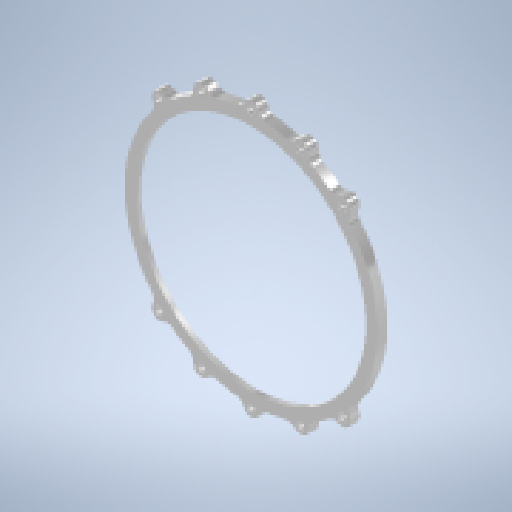
# Autodesk Inventor part: 出力ベアリング抑え
Saved by Autodesk Inventor 2024 (Build 280153000, 153)
## iProperties
Created: 2023-05-29
Part Number: 出力ベアリング抑え
Material: アルミニウム 6061
Document SubType Name: Modeling
Designer: yuta2
Density: 2.7 g/cm^3
Appearance: アルミニウム - フラット
Author: yuta2
Autodesk Inventor part; units mm, degrees
ref_plane "YZ Plane" through (0, 0, 0) normal (1, 0, 0) x (0, 1, 0)
ref_plane "XZ Plane" through (0, 0, 0) normal (0, 1, 0) x (-1, 0, 0)
ref_plane "XY Plane" through (0, 0, 0) normal (0, 0, 1) x (1, 0, 0)
sketch "スケッチ1" plane through (0, 0, 0) normal (0, 0, 1) x (1, 0, 0)
  circle A0 centre (0, 0) radius 59
  circle A1 centre (0, 0) radius 65
  dimension "d0" = 118
  dimension "d1" = 130
  constraints: 2 centre point, 2 coincident
  measures "d0" diameter of A0
  measures "d1" diameter of A1
extrude "押し出し1" add sketch "スケッチ1" along normal blind 2.5
sketch "スケッチ2" plane through (0, 0, 0) normal (0, 0, -1) x (-1, 0, 0)
  circle A0 centre (0, 0) radius 65 projected
  circle A1 centre (0, 0) radius 59 projected
  circle A2 centre (0, 0) radius 62.5
  dimension "d4" = 125
  constraints: 1 centre point, 1 coincident
  measures "d4" diameter of A2
extrude "押し出し2" add sketch "スケッチ2" along normal blind 2.5 contours A0
sketch "スケッチ3" plane through (0, 0, 2.5) normal (0, 0, 1) x (1, 0, 0)
  circle A0 centre (0, 0) radius 65 projected
  circle A1 centre (0, 0) radius 62.5 projected
  circle A2 centre (0, 66.5) radius 4
  point P0 (3.6646, 64.8966)
  point P1 (-3.6646, 64.8966)
  dimension "d7" = 8
  constraints: 1 centre point, 1 tangent, 1 vertical alignment
  measures "d7" diameter of A2
extrude "押し出し3" add sketch "スケッチ3" against normal blind 5 contours A0 A2 picked at (-0.1169, 66.8205)
fillet "フィレット1" radius 5 4 edges at (3.6646, 64.8966, 1.25) (3.6646, 64.8966, -1.25) (-3.6646, 64.8966, 1.25) (-3.6646, 64.8966, -1.25)
pattern_circular "円形状パターン1" count 16 over 360 about axis through (0, 0, 0) along (0, 0, 1) of "押し出し3", "フィレット1"
sketch "スケッチ4" plane through (0, 0, 2.5) normal (0, 0, 1) x (1, 0, 0)
  arc A0 (-7.8847, 64.52) -> (-17.4062, 62.6261) centre (0, 0) ccw projected
  arc A1 (-22.4692, 64.1071) -> (-17.4062, 62.6261) centre (-18.7451, 67.4435) ccw projected
  arc A2 (-22.4692, 64.1071) -> (-29.4424, 61.2187) centre (-25.4484, 61.438) ccw projected
  arc A3 (-31.9753, 56.5914) -> (-29.4424, 61.2187) centre (-34.4349, 60.9445) ccw projected
  arc A4 (-31.9753, 56.5914) -> (-40.0472, 51.1979) centre (0, 0) ccw projected
  arc A5 (-45.2916, 50.6286) -> (-40.0472, 51.1979) centre (-43.1277, 55.1362) ccw projected
  arc A6 (-45.2916, 50.6286) -> (-50.6286, 45.2916) centre (-47.0226, 47.0226) ccw projected
  arc A7 (-51.1979, 40.0472) -> (-50.6286, 45.2916) centre (-55.1362, 43.1277) ccw projected
  arc A8 (-51.1979, 40.0472) -> (-56.5914, 31.9753) centre (0, 0) ccw projected
  arc A9 (-61.2187, 29.4424) -> (-56.5914, 31.9753) centre (-60.9445, 34.4349) ccw projected
  arc A10 (-61.2187, 29.4424) -> (-64.1071, 22.4692) centre (-61.438, 25.4484) ccw projected
  arc A11 (-62.6261, 17.4062) -> (-64.1071, 22.4692) centre (-67.4435, 18.7451) ccw projected
  arc A12 (-62.6261, 17.4062) -> (-64.52, 7.8847) centre (0, 0) ccw projected
  arc A13 (-67.8258, 3.7739) -> (-64.52, 7.8847) centre (-69.4831, 8.4912) ccw projected
  arc A14 (-67.8258, 3.7739) -> (-67.8258, -3.7739) centre (-66.5, 0) ccw projected
  arc A15 (-64.52, -7.8847) -> (-67.8258, -3.7739) centre (-69.4831, -8.4912) ccw projected
  arc A16 (-64.52, -7.8847) -> (-62.6261, -17.4062) centre (0, 0) ccw projected
  arc A17 (-64.1071, -22.4692) -> (-62.6261, -17.4062) centre (-67.4435, -18.7451) ccw projected
  arc A18 (-64.1071, -22.4692) -> (-61.2187, -29.4424) centre (-61.438, -25.4484) ccw projected
  arc A19 (-56.5914, -31.9753) -> (-61.2187, -29.4424) centre (-60.9445, -34.4349) ccw projected
  arc A20 (-56.5914, -31.9753) -> (-51.1979, -40.0472) centre (0, 0) ccw projected
  arc A21 (-50.6286, -45.2916) -> (-51.1979, -40.0472) centre (-55.1362, -43.1277) ccw projected
  arc A22 (-50.6286, -45.2916) -> (-45.2916, -50.6286) centre (-47.0226, -47.0226) ccw projected
  arc A23 (-40.0472, -51.1979) -> (-45.2916, -50.6286) centre (-43.1277, -55.1362) ccw projected
  arc A24 (-40.0472, -51.1979) -> (-31.9753, -56.5914) centre (0, 0) ccw projected
  arc A25 (-29.4424, -61.2187) -> (-31.9753, -56.5914) centre (-34.4349, -60.9445) ccw projected
  arc A26 (-29.4424, -61.2187) -> (-22.4692, -64.1071) centre (-25.4484, -61.438) ccw projected
  arc A27 (-17.4062, -62.6261) -> (-22.4692, -64.1071) centre (-18.7451, -67.4435) ccw projected
  arc A28 (-17.4062, -62.6261) -> (-7.8847, -64.52) centre (0, 0) ccw projected
  arc A29 (-3.7739, -67.8258) -> (-7.8847, -64.52) centre (-8.4912, -69.4831) ccw projected
  arc A30 (-3.7739, -67.8258) -> (3.7739, -67.8258) centre (0, -66.5) ccw projected
  arc A31 (7.8847, -64.52) -> (3.7739, -67.8258) centre (8.4912, -69.4831) ccw projected
  arc A32 (7.8847, -64.52) -> (17.4062, -62.6261) centre (0, 0) ccw projected
  arc A33 (22.4692, -64.1071) -> (17.4062, -62.6261) centre (18.7451, -67.4435) ccw projected
  arc A34 (22.4692, -64.1071) -> (29.4424, -61.2187) centre (25.4484, -61.438) ccw projected
  arc A35 (31.9753, -56.5914) -> (29.4424, -61.2187) centre (34.4349, -60.9445) ccw projected
  arc A36 (31.9753, -56.5914) -> (40.0472, -51.1979) centre (0, 0) ccw projected
  arc A37 (45.2916, -50.6286) -> (40.0472, -51.1979) centre (43.1277, -55.1362) ccw projected
  arc A38 (45.2916, -50.6286) -> (50.6286, -45.2916) centre (47.0226, -47.0226) ccw projected
  arc A39 (51.1979, -40.0472) -> (50.6286, -45.2916) centre (55.1362, -43.1277) ccw projected
  arc A40 (51.1979, -40.0472) -> (56.5914, -31.9753) centre (0, 0) ccw projected
  arc A41 (61.2187, -29.4424) -> (56.5914, -31.9753) centre (60.9445, -34.4349) ccw projected
  arc A42 (61.2187, -29.4424) -> (64.1071, -22.4692) centre (61.438, -25.4484) ccw projected
  arc A43 (62.6261, -17.4062) -> (64.1071, -22.4692) centre (67.4435, -18.7451) ccw projected
  arc A44 (62.6261, -17.4062) -> (64.52, -7.8847) centre (0, 0) ccw projected
  arc A45 (67.8258, -3.7739) -> (64.52, -7.8847) centre (69.4831, -8.4912) ccw projected
  arc A46 (67.8258, -3.7739) -> (67.8258, 3.7739) centre (66.5, 0) ccw projected
  arc A47 (64.52, 7.8847) -> (67.8258, 3.7739) centre (69.4831, 8.4912) ccw projected
  arc A48 (64.52, 7.8847) -> (62.6261, 17.4062) centre (0, 0) ccw projected
  arc A49 (64.1071, 22.4692) -> (62.6261, 17.4062) centre (67.4435, 18.7451) ccw projected
  arc A50 (64.1071, 22.4692) -> (61.2187, 29.4424) centre (61.438, 25.4484) ccw projected
  arc A51 (56.5914, 31.9753) -> (61.2187, 29.4424) centre (60.9445, 34.4349) ccw projected
  arc A52 (56.5914, 31.9753) -> (51.1979, 40.0472) centre (0, 0) ccw projected
  arc A53 (50.6286, 45.2916) -> (51.1979, 40.0472) centre (55.1362, 43.1277) ccw projected
  arc A54 (50.6286, 45.2916) -> (45.2916, 50.6286) centre (47.0226, 47.0226) ccw projected
  arc A55 (40.0472, 51.1979) -> (45.2916, 50.6286) centre (43.1277, 55.1362) ccw projected
  arc A56 (40.0472, 51.1979) -> (31.9753, 56.5914) centre (0, 0) ccw projected
  arc A57 (29.4424, 61.2187) -> (31.9753, 56.5914) centre (34.4349, 60.9445) ccw projected
  arc A58 (29.4424, 61.2187) -> (22.4692, 64.1071) centre (25.4484, 61.438) ccw projected
  arc A59 (17.4062, 62.6261) -> (22.4692, 64.1071) centre (18.7451, 67.4435) ccw projected
  arc A60 (17.4062, 62.6261) -> (7.8847, 64.52) centre (0, 0) ccw projected
  arc A61 (3.7739, 67.8258) -> (7.8847, 64.52) centre (8.4912, 69.4831) ccw projected
  arc A62 (3.7739, 67.8258) -> (-3.7739, 67.8258) centre (0, 66.5) ccw projected
  arc A63 (-7.8847, 64.52) -> (-3.7739, 67.8258) centre (-8.4912, 69.4831) ccw projected
  circle A64 centre (0, 0) radius 59 projected
  circle A65 centre (0, 0) radius 65
  point P0 (62.6261, -17.4062)
  point P1 (56.5914, -31.9753)
  point P2 (64.52, 7.8847)
  point P3 (64.52, -7.8847)
  point P4 (56.5914, 31.9753)
  point P5 (62.6261, 17.4062)
  point P6 (-56.5914, -31.9753)
  point P7 (-62.6261, -17.4062)
  point P8 (-64.52, -7.8847)
  point P9 (-64.52, 7.8847)
  point P10 (-62.6261, 17.4062)
  constraints: 1 centre point, 1 coincident, 1 concentric
extrude "押し出し4" cut sketch "スケッチ4" against normal through all contours A65 A11 A10 A9 | A51 A50 A49 A65 | A65 A15 A14 A13 | A47 A46 A45 A65 | A65 A19 A18 A17 | A43 A42 A41 A65
sketch "スケッチ5" plane through (0, 0, 2.5) normal (0, 0, 1) x (1, 0, 0)
  arc A0 (-45.2916, 50.6286) -> (-50.6286, 45.2916) centre (-47.0226, 47.0226) ccw projected
  arc A1 (-22.4692, 64.1071) -> (-29.4424, 61.2187) centre (-25.4484, 61.438) ccw projected
  arc A2 (3.7739, 67.8258) -> (-3.7739, 67.8258) centre (0, 66.5) ccw projected
  arc A3 (29.4424, 61.2187) -> (22.4692, 64.1071) centre (25.4484, 61.438) ccw projected
  arc A4 (50.6286, 45.2916) -> (45.2916, 50.6286) centre (47.0226, 47.0226) ccw projected
  arc A5 (45.2916, -50.6286) -> (50.6286, -45.2916) centre (47.0226, -47.0226) ccw projected
  arc A6 (22.4692, -64.1071) -> (29.4424, -61.2187) centre (25.4484, -61.438) ccw projected
  arc A7 (-3.7739, -67.8258) -> (3.7739, -67.8258) centre (0, -66.5) ccw projected
  arc A8 (-29.4424, -61.2187) -> (-22.4692, -64.1071) centre (-25.4484, -61.438) ccw projected
  arc A9 (-50.6286, -45.2916) -> (-45.2916, -50.6286) centre (-47.0226, -47.0226) ccw projected
  point P0 (0, 0)
  constraints: 10 coincident
hole "穴1" at (-47.0226, 47.0226, 2.5) at (-25.4484, 61.438, 2.5) at (0, 66.5, 2.5) at (25.4484, 61.438, 2.5) at (47.0226, 47.0226, 2.5) at (47.0226, -47.0226, 2.5) at (25.4484, -61.438, 2.5) at (0, -66.5, 2.5) at (-25.4484, -61.438, 2.5) at (-47.0226, -47.0226, 2.5) direction (0, 0, -1) diameter 4.1 end through all
